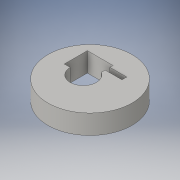
# Autodesk Inventor part: top hook
Saved by Autodesk Inventor 2016 (Build 200138000, 138)
## iProperties
Created: 2016-01-16
Part Number: top hook
Material: Generic
Document SubType Name: Modeling
Designer: Administrator
Density: 1 g/cm^3
Appearance: Default
Author: Administrator
Autodesk Inventor part; units mm, degrees
ref_plane "YZ Plane" through (0, 0, 0) normal (1, 0, 0) x (0, 1, 0)
ref_plane "XZ Plane" through (0, 0, 0) normal (0, 1, 0) x (-1, 0, 0)
ref_plane "XY Plane" through (0, 0, 0) normal (0, 0, 1) x (1, 0, 0)
sketch "Sketch1" plane through (0, 0, 0) normal (0, 1, 0) x (-1, 0, 0)
  circle A0 centre (0, 0) radius 12.7
  dimension "d0" = 25.4
  constraints: 1 centre point, 1 coincident
  measures "d0" diameter of A0
extrude "Extrusion1" add sketch "Sketch1" along normal blind 5.8674
sketch "Sketch2" plane through (0, 5.8674, 0) normal (0, 1, 0) x (1, 0, 0)
  line L0 (0, 0) -> (-7.7692, 0)
  line L1 (-7.7692, 0) -> (-7.7692, 6.975)
  line L2 (-7.7692, 6.975) -> (0, 6.975)
  line L3 (0, 6.975) -> (0, 0)
  constraints: 8 end point, 2 parallel, 1 horizontal, 1 perpendicular
extrude "Extrusion2" cut sketch "Sketch2" against normal blind 254
sketch "Sketch3" plane through (0, 5.8674, 0) normal (0, 1, 0) x (1, 0, 0)
  line L0 (0, 6.018) -> (5.0945, 6.018)
  line L1 (5.0945, 6.018) -> (5.0945, 4.5769)
  line L2 (5.0945, 4.5769) -> (0, 4.5769)
  line L3 (0, 4.5769) -> (0, 6.018)
  point P0 (0, 0)
  constraints: 8 end point, 2 parallel, 1 horizontal, 1 perpendicular
extrude "Extrusion3" cut sketch "Sketch3" against normal blind 254
sketch "Sketch4" plane through (0, 5.8674, 0) normal (0, 1, 0) x (1, 0, 0)
  circle A0 centre (-2.0297, 0) radius 3.9608
  point P0 (0, 0)
  constraints: 1 centre point
extrude "Extrusion4" cut sketch "Sketch4" against normal blind 254
body "Solid1"
